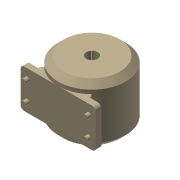
# Autodesk Inventor part: Motor1
Saved by Autodesk Inventor 2022.5 (Build 265521000, 521)
## iProperties
Created: 2015-09-08
Part Number: Motor1
Document SubType Name: Modeling
Designer: Administrator
Density: 1 g/cm^3
Mass: 6.40148 g
Surface Area: 22.6354 cm^2
Volume: 6.40148 cm^3
Material: Generic
Appearance: Beige
Author: Administrator
Autodesk Inventor part; units mm, degrees
ref_plane "YZ Plane" through (0, 0, 0) normal (1, 0, 0) x (0, 1, 0)
ref_plane "XZ Plane" through (0, 0, 0) normal (0, 1, 0) x (-1, 0, 0)
ref_plane "XY Plane" through (0, 0, 0) normal (0, 0, 1) x (1, 0, 0)
sketch "Sketch1" plane through (0, 0, 0) normal (0, 0, 1) x (1, 0, 0)
  circle A0 centre (0, 0) radius 17.5
  dimension "d0" = 35
  constraints: 1 centre point, 1 other
  measures "d0" diameter of A0
extrude "Extrusion1" add sketch "Sketch1" along normal mid plane 30
sketch "Sketch2" plane through (0, 0, 0) normal (0, 0, 1) x (1, 0, 0)
  line L0 (0, 0) -> (0, -17.5) construction
  line L1 (0, -17.5) -> (-17.5, -17.5)
  line L2 (-17.5, -17.5) -> (-17.5, -14.5) construction
  line L3 (-17.5, -14.5) -> (-13.5, -14.5)
  line L4 (-13.5, -14.5) -> (-11.1906, -10.5)
  line L5 (0, -17.5) -> (17.5, -17.5)
  line L6 (17.5, -17.5) -> (17.5, -14.5) construction
  line L7 (17.5, -14.5) -> (13.5, -14.5)
  line L8 (13.5, -14.5) -> (11.1906, -10.5)
  line L9 (-11.1906, -10.5) -> (11.1906, -10.5)
  circle A0 centre (0, 0) radius 17.5 construction
  line L10 (0, 0) -> (0, -17.5) construction
  line L11 (0, -17.5) -> (25.1989, -17.5) construction
  line L12 (0, 0) -> (-17.5, 0) construction
  line L13 (-17.5, -14.5) -> (-19.5, -14.5)
  line L14 (-19.5, -14.5) -> (-19.5, -17.5)
  line L15 (-19.5, -17.5) -> (-17.5, -17.5)
  line L16 (17.5, -14.5) -> (19.5, -14.5)
  line L17 (19.5, -14.5) -> (19.5, -17.5)
  line L18 (19.5, -17.5) -> (17.5, -17.5)
  dimension "d4" = 3
  dimension "d5" = 4
  dimension "d6" = 60
  dimension "d16" = 0
  dimension "d17" = 4
  dimension "d18" = 2
  dimension "d31" = 35
  dimension "d32" = 39
  constraints: 38 end point, 6 perpendicular, 4 symmetric about line, 3 horizontal, 2 equal length, 2 parallel, 2 point on circle, 2 vertical, 1 collinear, 1 tangent
  measures "d4" distance between parallel lines of L3 L1
  measures "d5" distance of L2.end L3.end
  measures "d6" angle of L4 L3
  measures "d16" distance between parallel lines of L5 L11
  measures "d17" distance between parallel lines of L9 L7
  measures "d18" distance of L2.end L13.end
  measures "d31" diameter of A0
  measures "d32" distance between parallel lines of L17 L14
extrude "Extrusion2" add sketch "Sketch2" along normal mid plane 20
chamfer "Chamfer1" distance 3 angle 45 2 edges at (-17.5, 0, 15) (-17.5, 0, -15)
sketch "Sketch3" plane through (0, 0, 15) normal (0, 0, 1) x (1, 0, 0)
  circle A0 centre (0, 0) radius 14.5 projected
  circle A1 centre (0, 0) radius 3
  dimension "d12" = 6
  constraints: 1 centre point
  measures "d12" diameter of A1
extrude "Extrusion3" cut sketch "Sketch3" against normal blind 8 contours A1
sketch "Sketch4" plane through (-19.5, -17.5, 10) normal (0, -1, 0) x (1, 0, 0)
  line L0 (19.5, 0) -> (0, 0) construction
  line L1 (0, 0) -> (0, -20) construction
  line L2 (0, -20) -> (19.5, -20) construction
  line L3 (39, 0) -> (39, -20) construction
  line L4 (2, -22) -> (2, 2) construction
  line L5 (37, -22) -> (37, 2) construction
  line L6 (33, 0) -> (33, -20) construction
  line L7 (7.1902, -20) -> (7.1902, 0) construction
  line L8 (2, -5) -> (37, -5) construction
  line L9 (37, -5) -> (37, -15) construction
  line L10 (37, -15) -> (2, -15) construction
  line L11 (2, -15) -> (2, -5) construction
  line L12 (19.5, -20) -> (39, -20) projected
  line L13 (39, 0) -> (19.5, 0) projected
  line L14 (19.5, -20) -> (31.8098, -20) construction
  line L15 (19.5, -20) -> (19.5, 0) construction
  line L16 (22.5, -3) -> (16.5, -3) construction
  line L17 (3.5, -5) -> (35.5, -5) construction
  line L18 (35.5, -5) -> (35.5, -15) construction
  line L19 (35.5, -15) -> (3.5, -15) construction
  line L20 (3.5, -15) -> (3.5, -5) construction
  circle A0 centre (3.5, -5) radius 1.25
  circle A1 centre (3.5, -15) radius 1.25
  circle A2 centre (35.5, -5) radius 1.25
  circle A3 centre (35.5, -15) radius 1.25
  point P0 (19.5, -10)
  dimension "d19" = 5
  dimension "d20" = 5
  dimension "d33" = 16
  dimension "d34" = 16
  dimension "d35" = 2.5
  constraints: 18 end point, 4 centre point, 4 coincident, 4 parallel, 4 point on line, 3 equal radius, 3 perpendicular, 2 horizontal
  measures "d19" distance between parallel lines of L0 L8
  measures "d20" distance between parallel lines of L10 L2
  measures "d33" distance between parallel lines of L20 L15
  measures "d34" distance between parallel lines of L18 L15
  measures "d35" diameter of A1
extrude "Extrusion4" cut sketch "Sketch4" against normal up to surface (3 mm away)
fillet "Fillet2" radius 2 4 edges at (-19.5, -16, 10) (19.5, -16, 10) (19.5, -16, -10) (-19.5, -16, -10)
sketch "Sketch5" plane through (-13.5, -14.5, 10) normal (0, 1, 0) x (1, 0, 0)
  arc A0 (-4, 20) -> (-6, 18) centre (-4, 18) ccw projected
  line L0 (-6, 2) -> (-6, 18) projected
  arc A1 (-6, 2) -> (-4, 0) centre (-4, 2) ccw projected
  line L1 (-4, 0) -> (0, 0) projected
  line L2 (0, 0) -> (0, 20) projected
  line L3 (0, 20) -> (-4, 20) projected
  line L4 (31.5, 3.8453) -> (29.5, 2.6906)
  line L5 (29.5, 2.6906) -> (27.5, 3.8453)
  line L6 (27.5, 3.8453) -> (27.5, 6.1547)
  line L7 (27.5, 6.1547) -> (29.5, 7.3094)
  line L8 (29.5, 7.3094) -> (31.5, 6.1547)
  line L9 (31.5, 6.1547) -> (31.5, 3.8453)
  circle A2 centre (-2.5, 5) radius 1.25 projected
  circle A3 centre (-2.5, 15) radius 1.25 projected
  circle A4 centre (29.5, 5) radius 1.25 projected
  circle A5 centre (29.5, 15) radius 1.25 projected
  line L10 (-6, 2) -> (-6, 18) projected
  line L11 (27.5, 13.8453) -> (27.5, 16.1547)
  line L12 (29.5, 12.6906) -> (27.5, 13.8453)
  line L13 (27.5, 16.1547) -> (29.5, 17.3094)
  line L14 (29.5, 17.3094) -> (31.5, 16.1547)
  line L15 (31.5, 16.1547) -> (31.5, 13.8453)
  line L16 (31.5, 13.8453) -> (29.5, 12.6906)
  line L17 (-4.5, 13.8453) -> (-4.5, 16.1547)
  line L18 (-2.5, 12.6906) -> (-4.5, 13.8453)
  line L19 (-4.5, 16.1547) -> (-2.5, 17.3094)
  line L20 (-2.5, 17.3094) -> (-0.5, 16.1547)
  line L21 (-0.5, 16.1547) -> (-0.5, 13.8453)
  line L22 (-0.5, 13.8453) -> (-2.5, 12.6906)
  line L23 (-4.5, 3.8453) -> (-4.5, 6.1547)
  line L24 (-2.5, 2.6906) -> (-4.5, 3.8453)
  line L25 (-4.5, 6.1547) -> (-2.5, 7.3094)
  line L26 (-2.5, 7.3094) -> (-0.5, 6.1547)
  line L27 (-0.5, 6.1547) -> (-0.5, 3.8453)
  line L28 (-0.5, 3.8453) -> (-2.5, 2.6906)
  point P0 (13.5, 10)
  dimension "d26" = 4
  dimension "d36" = 4
  dimension "d37" = 4
  dimension "d38" = 4
  constraints: 48 end point, 4 coincident, 52 other
  measures "d26" distance between parallel lines of L6 L9
  measures "d36" distance between parallel lines of L11 L15
  measures "d37" distance between parallel lines of L17 L21
  measures "d38" distance between parallel lines of L23 L27
extrude "Extrusion5" add sketch "Sketch5" along normal blind 1.5 contours L4 L5 L6 L7 L8 L9 | A2 | A3 | A4 | A5 | L11 L13 L14 L15 L16 L12 | L17 L19 L20 L21 L22 L18 | L23 L25 L26 L27 L28 L24
sketch "Sketch6" plane through (-17.5, -17.5, -10) normal (0, -1, 0) x (1, 0, 0)
  circle A0 centre (1.5, 15) radius 1.25 projected
  circle A1 centre (33.5, 15) radius 1.25 projected
  circle A2 centre (1.5, 5) radius 1.25 projected
  circle A3 centre (33.5, 5) radius 1.25 projected
  point P0 (17.5, 10)
extrude "Extrusion6" add sketch "Sketch6" along normal mid plane 4
body "Solid1"
